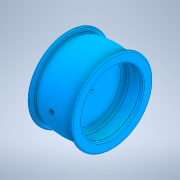
# Autodesk Inventor part: Toe
Saved by Autodesk Inventor 2022.2 (Build 262287000, 287)
## iProperties
Created: 2021-12-28
Part Number: Toe
Material: Generic
Document SubType Name: Modeling
Designer: Jochen
Density: 1 g/cm^3
Appearance: Default
Author: Jochen
Autodesk Inventor part; units mm, degrees
ref_plane "YZ Plane" through (0, 0, 0) normal (1, 0, 0) x (0, 1, 0)
ref_plane "XZ Plane" through (0, 0, 0) normal (0, 1, 0) x (-1, 0, 0)
sketch "ToeSketch" plane through (0, 0, 0) normal (0, 0, 1) x (1, 0, 0)
  line L0 (-11.666, 0) -> (11.666, 0) construction
  line L1 (0, -16.1502) -> (0, 19.9967) construction
  line L2 (-8.25, 12.3131) -> (-8.25, 11.6707)
  line L3 (8.25, 12.3131) -> (8.25, 11.6707)
  line L4 (0.75, 0.625) -> (0.75, 10.5)
  line L5 (0.75, 0.625) -> (-0.75, 0.625)
  line L6 (-0.75, 0.625) -> (-0.75, 10.5)
  line L7 (-7.85, 11.2707) -> (-7.1375, 11.2707)
  arc A0 (-2.8705, 11.5882) -> (-6.8566, 11.3859) centre (-4.75, 9.25) ccw
  arc A1 (6.8566, 11.3859) -> (2.8705, 11.5882) centre (4.75, 9.25) ccw
  line L8 (7.1375, 11.2707) -> (7.85, 11.2707)
  line L9 (-2.6199, 11.5) -> (-1.75, 11.5)
  line L10 (1.75, 11.5) -> (2.6199, 11.5)
  arc A2 (7.85, 11.2707) -> (8.25, 11.6707) centre (7.85, 11.6707) ccw
  arc A3 (8.25, 12.3131) -> (7.9777, 12.6922) centre (7.85, 12.3131) ccw
  arc A4 (-8.25, 11.6707) -> (-7.85, 11.2707) centre (-7.85, 11.6707) ccw
  arc A5 (-7.1375, 11.2707) -> (-6.8566, 11.3859) centre (-7.1375, 11.6707) ccw
  arc A6 (6.8566, 11.3859) -> (7.1375, 11.2707) centre (7.1375, 11.6707) ccw
  arc A7 (6.3927, 13.1684) -> (-6.3927, 13.1684) centre (0, -10.9864) ccw
  arc A8 (-2.8705, 11.5882) -> (-2.6199, 11.5) centre (-2.6199, 11.9) ccw
  arc A9 (2.6199, 11.5) -> (2.8705, 11.5882) centre (2.6199, 11.9) ccw
  arc A10 (-0.75, 10.5) -> (-1.75, 11.5) centre (-1.75, 10.5) ccw
  arc A11 (1.75, 11.5) -> (0.75, 10.5) centre (1.75, 10.5) ccw
  circle A12 centre (-4.75, 9.25) radius 3 construction
  circle A13 centre (4.75, 9.25) radius 3 construction
  line L11 (5.4355, 12.1706) -> (5.7098, 13.3389) construction
  line L12 (7.9777, 12.6922) -> (7.4988, 11.2707) construction
  line L13 (-7.2, 11.2707) -> (-7.2, 10.6)
  line L14 (-6.4, 9.8) -> (6.4, 9.8)
  line L15 (7.2, 10.6) -> (7.2, 11.2707)
  arc A14 (6.4, 9.8) -> (7.2, 10.6) centre (6.4, 10.6) ccw
  arc A15 (-7.2, 10.6) -> (-6.4, 9.8) centre (-6.4, 10.6) ccw
  line L16 (8.25, 12.3131) -> (8.25, 14.35)
  line L17 (7.85, 14.75) -> (7.55, 14.75)
  line L18 (-8.25, 12.3131) -> (-8.25, 14.35)
  line L19 (-7.85, 14.75) -> (-7.55, 14.75)
  arc A16 (8.25, 14.35) -> (7.85, 14.75) centre (7.85, 14.35) ccw
  arc A17 (7.55, 14.75) -> (7.165, 14.4584) centre (7.55, 14.35) ccw
  arc A18 (-7.165, 14.4584) -> (-7.55, 14.75) centre (-7.55, 14.35) ccw
  arc A19 (-7.85, 14.75) -> (-8.25, 14.35) centre (-7.85, 14.35) ccw
  arc A20 (-6.8801, 13.4466) -> (-6.3927, 13.1684) centre (-6.495, 13.5551) ccw
  arc A21 (6.3927, 13.1684) -> (6.8801, 13.4466) centre (6.495, 13.5551) ccw
  line L20 (-7.165, 14.4584) -> (-6.8801, 13.4466)
  line L21 (6.8801, 13.4466) -> (7.165, 14.4584)
  point P0 (0, 0)
  point P1 (-8.25, 10.6859)
  point P2 (8.25, 10.6859)
  point P3 (8.25, 11.2707)
  point P4 (-6.9674, 11.2707)
  point P5 (-2.7657, 11.5)
  point P6 (2.7657, 11.5)
  point P7 (0, 14)
  point P8 (6.9674, 11.2707)
  point P9 (0.75, 11.5)
  point P10 (8.238, 12.0321)
  point P11 (-7.2, 9.8)
  point P12 (7.2, 9.8)
  point P13 (-0.75, 9.8)
  point P14 (0.75, 9.8)
  point P15 (7.0882, 14.1857)
  dimension "d2" = 1.5
  dimension "d3" = 0.625
  dimension "d9" = 0.4
  dimension "d11" = 16.5
  dimension "d12" = 11.5
  dimension "d19" = 1
  dimension "d21" = 3
  dimension "d24" = 9.25
  dimension "d25" = 14
  dimension "d27" = 1.2
  dimension "d30" = 9.8
  dimension "d32" = 14.4
  dimension "d33" = 0.8
  dimension "d54" = 9.5
  dimension "d57" = 0.75
  dimension "d58" = 0.3
  constraints: 46 point on circle, 40 end point, 34 tangent, 21 centre point, 19 point on line, 13 equal radius, 8 perpendicular, 5 line through centre, 4 horizontal, 4 vertical, 3 collinear, 2 coincident, 1 concentric, 11 other
  measures "d2" distance between parallel lines of L4 L6
  measures "d3" distance from line of L4.start L0
  measures "d9" radius of A2
  measures "d11" distance between parallel lines of L3 L2
  measures "d12" distance between parallel lines of L0 L10
  measures "d19" radius of A10
  measures "d21" radius of A1
  measures "d24" distance from line of L0 A1.centre
  measures "d25" distance from line of L0 point (0, 14)
  measures "d27" distance of L11.start L11.end
  measures "d30" distance between parallel lines of L0 L14
  measures "d32" distance of point (-7.2, 9.8) point (7.2, 9.8)
  measures "d33" radius of A14
  measures "d54" distance of point (4.75, 9.25) A0.centre
  measures "d57" distance edge to line of A7 L17
  measures "d58" distance of L17.start L17.end
revolve "Revolution2" [suppressed]
sketch "Sketch2" plane through (0, 0, 0) normal (1, 0, 0) x (0, 1, 0)
  line L0 (16.0374, -3.8798) -> (16.0374, 3.8798)
  circle A0 centre (0, 0) radius 16.5
  line L1 (-23.1, 0) -> (23.1, 0) construction
  line L2 (0, -23.1) -> (0, 23.1) construction
  line L3 (16.0374, 3.8798) -> (-16.5, 0)
  line L4 (16.0374, -3.8798) -> (-16.5, 0)
  line L5 (11.3787, -11.9488) -> (-8.25, 14.2894)
  line L6 (4.6586, -15.8287) -> (-8.25, 14.2894)
  line L7 (-4.6586, -15.8287) -> (8.25, 14.2894)
  line L8 (-11.3787, -11.9488) -> (8.25, 14.2894)
  line L9 (-16.0374, -3.8798) -> (16.5, 0)
  line L10 (-16.0374, 3.8798) -> (16.5, 0)
  line L11 (-11.3787, 11.9488) -> (8.25, -14.2894)
  line L12 (-4.6586, 15.8287) -> (8.25, -14.2894)
  line L13 (4.6586, 15.8287) -> (-8.25, -14.2894)
  line L14 (11.3787, 11.9488) -> (-8.25, -14.2894)
  point P0 (0, 4.9593)
  point P1 (-4.2949, 2.4796)
  point P2 (-11.3787, 11.9488)
  point P3 (-4.2949, -2.4796)
  point P4 (-16.0374, -3.8798)
  point P5 (-11.3787, -11.9488)
  point P6 (0, -4.9593)
  point P7 (-4.6586, -15.8287)
  point P8 (4.6586, -15.8287)
  point P9 (4.2949, 2.4796)
  point P10 (4.2949, -2.4796)
  point P11 (11.3787, -11.9488)
  point P12 (-1.2199, -2.113)
  point P13 (-1.2199, 2.113)
  point P14 (-2.4399, 0)
  point P15 (2.4399, 0)
  point P16 (1.2199, -2.113)
  point P17 (1.2199, 2.113)
  dimension "d35" = 33
  dimension "d39" = 360
  dimension "d44" = 13.6
  constraints: 26 end point, 4 coincident, 4 point on circle, 1 centre point, 1 perpendicular, 1 point on line, 41 other
  measures "d35" diameter of A0
  measures "d44" angle of L4 L3
extrude "Extrusion1" [suppressed]
fillet "Fillet1" [suppressed]
revolve "Revolution1" add sketch "ToeSketch" angle 360 about axis through (-10, 0, 0) along (1, 0, 0) contours L18 A19 L19 A18 L20 A20 A7 A21 L21 A17 L17 A16 L16 L3 A2 L8 A6 A1 A9 L10 A11 L4 L14 L6 A10 L9 A8 A0 A5 L7 A4 L2 | L14 L4 L5 L6
ref_plane "Work Plane2" through (0, 0, 18) normal (0, 0, 1) x (1, 0, 0)
sketch "Sketch4" plane through (0, 0, 18) normal (0, 0, 1) x (1, 0, 0)
  line L0 (-11.55, 0) -> (11.55, 0) construction
  line L1 (0, -20.65) -> (0, 20.65) construction
  circle A0 centre (0, 0) radius 0.775
  line L2 (-1, 0) -> (1, 0) construction
  dimension "d46" = 1.55
  dimension "d47" = 1
  constraints: 4 end point, 1 centre point, 1 coincident, 1 midpoint, 1 point on line
  measures "d46" diameter of A0
  measures "d47" distance from line of L2.end L1
extrude "Extrusion2" cut sketch "Sketch4" against normal blind 7.5
body "Solid1"
body "Solid2"
